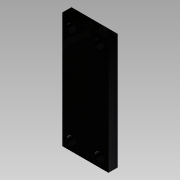
# Autodesk Inventor part: Plat
Saved by Autodesk Inventor 2015 SP1 (Build 190203100, 203)
## iProperties
Created: 2015-02-08
Part Number: Plat
Material: Generic
Document SubType Name: Modeling
Designer: Rafi Kurnia Putra
Density: 1 g/cm^3
Appearance: Smooth - Purple
Mass: 1.18717 g
Surface Area: 9.50531 cm^2
Volume: 1.18717 cm^3
Author: Rafi Kurnia Putra
Autodesk Inventor part; units mm, degrees
ref_plane "YZ Plane" through (0, 0, 0) normal (1, 0, 0) x (0, 1, 0)
ref_plane "XZ Plane" through (0, 0, 0) normal (0, 1, 0) x (-1, 0, 0)
ref_plane "XY Plane" through (0, 0, 0) normal (0, 0, 1) x (1, 0, 0)
sketch "Sketch1" plane through (0, 0, 0) normal (0, 1, 0) x (-1, 0, 0)
  line L0 (-12.5, 5) -> (12.5, 5)
  line L1 (12.5, 5) -> (12.5, -5)
  line L2 (12.5, -5) -> (-12.5, -5)
  line L3 (-12.5, -5) -> (-12.5, 5)
  circle A0 centre (10.5, 3) radius 1
  circle A1 centre (10.5, -3) radius 1
  circle A2 centre (-10.5, 3) radius 1
  circle A3 centre (-10.5, -3) radius 1
  point P0 (0, 0)
  point P1 (0, 0)
  dimension "d0" = 25
  dimension "d1" = 10
  dimension "d3" = 2
  dimension "d4" = 2
  dimension "d5" = 2
  dimension "d6" = 2
  dimension "d7" = 2
  dimension "d8" = 2
  dimension "d9" = 2
  dimension "d10" = 2
  dimension "d13" = 2
  dimension "d14" = 2
  dimension "d15" = 2
  dimension "d16" = 2
  dimension "d17" = 6
  dimension "d18" = 21
  constraints: 8 end point, 4 centre point, 2 parallel, 1 coincident, 1 horizontal, 1 perpendicular
  measures "d0" distance of L1.end L2.end
  measures "d1" distance of L0.end L1.end
  measures "d3" diameter of A0
  measures "d4" diameter of A1
  measures "d5" diameter of A2
  measures "d6" diameter of A3
  measures "d7" distance from line of A3.centre L3
  measures "d8" distance from line of A2.centre L3
  measures "d9" distance from line of A0.centre L1
  measures "d10" distance from line of A1.centre L1
  measures "d13" distance from line of A0.centre L0
  measures "d14" distance from line of L2 A1.centre
  measures "d15" distance from line of A2.centre L0
  measures "d16" distance from line of L2 A3.centre
  measures "d17" distance of A1.centre A0.centre
  measures "d18" distance of A3.centre A1.centre
extrude "Extrusion1" add sketch "Sketch1" along normal mid plane 2
body "Solid1"
